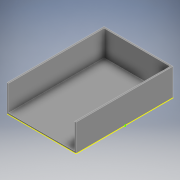
# Autodesk Inventor part: Part1
Saved by Autodesk Inventor 2021 (Build 250183000, 183)
## iProperties
Created: 2023-01-12
Part Number: Part1
Material: Generic
Document SubType Name: Modeling
Designer: boyle
Density: 1 g/cm^3
Appearance: Default
Author: boyle
Autodesk Inventor part; units mm, degrees
ref_plane "YZ Plane" through (0, 0, 0) normal (1, 0, 0) x (0, 1, 0)
ref_plane "XZ Plane" through (0, 0, 0) normal (0, 1, 0) x (-1, 0, 0)
ref_plane "XY Plane" through (0, 0, 0) normal (0, 0, 1) x (1, 0, 0)
sketch "Sketch1" plane through (0, 0, 0) normal (0, 1, 0) x (-1, 0, 0)
  line L0 (0, 0) -> (-177.8, 0)
  line L1 (-177.8, 0) -> (-177.8, 254)
  line L2 (-177.8, 254) -> (0, 254)
  line L3 (0, 254) -> (0, 0)
  dimension "d0" = 177.8
  dimension "d1" = 254
  constraints: 8 end point, 2 parallel, 1 horizontal, 1 perpendicular
  measures "d0" distance of L1.end L2.end
  measures "d1" distance of L0.end L1.end
extrude "Extrusion1" add sketch "Sketch1" along normal blind 69.85
shell "Shell1" thickness 3.81 removed faces 1 at (118.5333, 69.85, 169.3333)
sketch "Sketch2" plane through (0, 0, 254) normal (0, 0, 1) x (1, 0, 0)
  line L0 (0, 0) -> (177.8, 0) projected
  line L1 (177.8, 0) -> (177.8, 69.85) projected
  line L2 (0, 69.85) -> (177.8, 69.85) projected
  line L3 (0, 0) -> (0, 69.85) projected
extrude "Extrusion2" cut sketch "Sketch2" against normal up to surface (3.81 mm away)
sketch "Sketch3" plane through (0, 0, 0) normal (0, -1, 0) x (1, 0, 0)
  line L0 (177.8, 250.19) -> (0, 250.19) projected
  line L1 (0, 0) -> (0, 250.19) projected
  line L2 (177.8, 250.19) -> (177.8, 0) projected
  line L3 (177.8, 250.19) -> (0, 250.19) projected
  line L4 (0, 0) -> (0, 250.19) projected
  line L5 (177.8, 0) -> (0, 0) projected
  line L6 (177.8, 250.19) -> (177.8, 0) projected
  line L7 (177.8, 250.19) -> (177.8, 0) projected
  line L8 (0, 0) -> (0, 250.19) projected
  spline S0 degree 4 poles (177.8, 124.7066) (150.6939, 176.8475) (113.586, 16.2644) (38.413, 233.5705) (23.9233, 82.83) (0, 125.095) knots 0 0 0 0 0 0.526947 1 1 1 1 1
  point P0 (139.1985, 130.7231)
  point P1 (96.1464, 117.7224)
  point P2 (52.2761, 137.9834)
  point P3 (25.7676, 120.1193)
  point P4 (0, 125.095)
  point P5 (177.8, 124.7066)
  constraints: 1 midpoint, 1 point on line, 6 other
body "Solid1"
